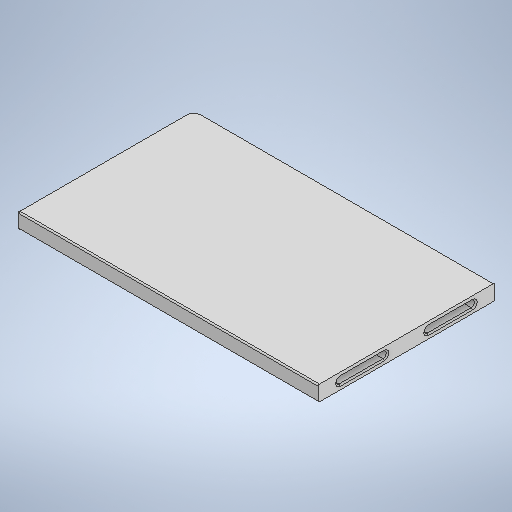
# Autodesk Inventor part: RighClamo3
Saved by Autodesk Inventor 2025.3 (Build 293356000, 356)
## iProperties
Created: 2025-11-20
Part Number: RighClamo3
Material: Generic
Document SubType Name: Modeling
Designer: User
Density: 1 g/cm^3
Appearance: Default
Author: User
Autodesk Inventor part; units mm, degrees
ref_plane "YZ Plane" through (0, 0, 0) normal (1, 0, 0) x (0, 1, 0)
ref_plane "XZ Plane" through (0, 0, 0) normal (0, 1, 0) x (-1, 0, 0)
ref_plane "XY Plane" through (0, 0, 0) normal (0, 0, 1) x (1, 0, 0)
sketch "Sketch1" plane through (0, 0, 0) normal (0, 1, 0) x (-1, 0, 0)
  line L0 (0, 0) -> (420, 0)
  line L1 (420, 0) -> (420, -40)
  line L2 (420, -40) -> (0, -40)
  line L3 (0, -40) -> (0, 0)
  dimension "d0" = 420
  dimension "d1" = 40
  constraints: 8 end point, 2 parallel, 1 horizontal, 1 perpendicular
  measures "d0" distance of L1.end L2.end
  measures "d1" distance of L0.end L1.end
extrude "Extrusion1" add sketch "Sketch1" along normal blind 3.5
fillet "Fillet1" radius 0.3 10 edges at (-210, 3.5, 0) (-210, 0, 0) (0, 0, -20) (0, 3.5, -20) (0, 1.75, -40) (-210, 3.5, -40) (-210, 0, -40) (-420, 0, -20) (-420, 1.75, -40) (-420, 3.5, -20)
sketch "Sketch2" plane through (0, 0, 0) normal (0, -1, 0) x (1, 0, 0)
  line L0 (-419.7, -39.7) -> (-419.7, -0.3) projected
  line L1 (-419.7, -20) -> (0, -20)
  circle A0 centre (-405, -20) radius 5
  circle A1 centre (-375, -20) radius 5
  circle A2 centre (-345, -20) radius 5
  circle A3 centre (-315, -20) radius 5
  line L2 (-420, 0) -> (-420, -39.7) projected
  line L3 (-315, -20) -> (-315, -8.0411)
  line L4 (-210.3, -20) -> (-630, -20)
  circle A4 centre (-225, -20) radius 5
  circle A5 centre (-255, -20) radius 5
  circle A6 centre (-285, -20) radius 5
  point P0 (0, 0)
  point P1 (-420, -0.3)
  dimension "d5" = 10
  dimension "d6" = 10
  dimension "d7" = 10
  dimension "d8" = 10
  dimension "d9" = 15
  dimension "d10" = 30
  dimension "d11" = 30
  dimension "d12" = 30
  constraints: 7 centre point, 7 point on line, 6 end point, 5 symmetric about line, 1 horizontal, 1 midpoint, 1 vertical, 3 other
  measures "d5" diameter of A0
  measures "d6" diameter of A1
  measures "d7" diameter of A2
  measures "d8" diameter of A3
  measures "d9" distance from line of L2 A0.centre
  measures "d10" distance of A1.centre A0.centre
  measures "d11" distance of A2.centre A1.centre
  measures "d12" distance of L3.start A2.centre
ref_plane "Work Plane1" through (-210, 0.3, -39.7) normal (1, 0, 0) x (0, 0, -1)
extrude "Extrusion2" cut sketch "Sketch2" against normal blind 3
mirror "Mirror1" about plane through (-210, 0.3, -39.7) normal (1, 0, 0) of "Extrusion2"
fillet "Fillet2" radius 2 6 edges at (-0.0879, 3.4121, -0.0879) (-0.0879, 0.0879, -0.0879) (0, 1.75, 0) (-419.9121, 3.4121, -0.0879) (-419.9121, 0.0879, -0.0879) (-420, 1.75, 0)
ref_plane "Work Plane2" through (-418, 0.3, -20) normal (0, 0, 1) x (1, 0, 0)
mirror "Mirror2" about plane through (-418, 0.3, -20) normal (0, 0, 1) remove original yes
sketch "Sketch3" plane through (-419.7, 3.5, -0.3) normal (0, 1, 0) x (1, 0, 0)
  line L0 (427.9018, 74.6307) -> (247.9018, 74.6307)
  line L1 (247.9018, 74.6307) -> (247.9018, -47.3259)
  line L2 (247.9018, -47.3259) -> (427.9018, -47.3259)
  line L3 (427.9018, -47.3259) -> (427.9018, 74.6307)
  line L4 (247.9018, 74.6307) -> (67.9018, 74.6307)
  line L5 (67.9018, 74.6307) -> (67.9018, -51.3741)
  line L6 (67.9018, -51.3741) -> (247.9018, -51.3741)
  line L7 (247.9018, -51.3741) -> (247.9018, 74.6307)
  line L8 (67.9018, 74.6307) -> (-27.6852, 74.6307)
  line L9 (-27.6852, 74.6307) -> (-27.6852, -51.3741)
  line L10 (-27.6852, -51.3741) -> (67.9018, -51.3741)
  line L11 (67.9018, -51.3741) -> (67.9018, 74.6307)
  point P0 (419.7, -0.3)
  point P1 (247.9018, -47.3259)
  point P2 (67.9018, -51.3741)
  point P3 (247.9018, -47.3259)
  dimension "d19" = 180
  dimension "d32" = 180
  constraints: 24 end point, 6 parallel, 3 horizontal, 3 perpendicular, 1 vertical
  measures "d19" distance of L0.start L0.end
  measures "d32" distance between parallel lines of L1 L5
extrude "Extrusion8" cut sketch "Sketch3" against normal through all contours L3 L2 L1 L0 | L1 L7 L6 L5 L4
sketch "Sketch7" plane through (-351.7982, 3.5, -0.3) normal (1, 0, 0) x (0, 0, -1)
  line L0 (4.7, -1.75) -> (14.7, -1.75) construction
  line L1 (4.7, -2.5) -> (14.7, -2.5)
  line L2 (14.7, -1) -> (4.7, -1)
  arc A0 (4.7, -1) -> (4.7, -2.5) centre (4.7, -1.75) ccw
  arc A1 (14.7, -2.5) -> (14.7, -1) centre (14.7, -1.75) ccw
  line L3 (24.7, -1.75) -> (34.7, -1.75) construction
  line L4 (24.7, -2.5) -> (34.7, -2.5)
  line L5 (34.7, -1) -> (24.7, -1)
  arc A2 (24.7, -1) -> (24.7, -2.5) centre (24.7, -1.75) ccw
  arc A3 (34.7, -2.5) -> (34.7, -1) centre (34.7, -1.75) ccw
  line L6 (39.7, -0.3) -> (39.7, -3.2) projected
  line L7 (-0.3, -3.2) -> (-0.3, -0.3) projected
  point P0 (-0.3, -3.5)
  point P1 (9.7, -1.75)
  point P2 (29.7, -1.75)
  dimension "d55" = 5
  dimension "d56" = 1.5
  dimension "d57" = 5
  dimension "d58" = 1.5
  dimension "d59" = 10
  dimension "d60" = 10
  constraints: 16 end point, 8 point on circle, 8 tangent, 4 centre point, 2 horizontal, 2 midpoint, 2 parallel
  measures "d55" distance of point (9.7, -1.75) L0.end
  measures "d56" diameter of A1
  measures "d57" distance of point (29.7, -1.75) L3.end
  measures "d58" diameter of A3
  measures "d59" distance from line of L6 point (29.7, -1.75)
  measures "d60" distance from line of L7 point (9.7, -1.75)
extrude "Extrusion9" cut sketch "Sketch7" against normal blind 16
chamfer "Chamfer3" distance 0.3 angle 45 8 edges at (-351.7982, 1.75, -15.75) (-351.7982, 1, -10) (-351.7982, 1.75, -4.25) (-351.7982, 2.5, -10) (-351.7982, 1.75, -24.25) (-351.7982, 2.5, -30) (-351.7982, 1.75, -35.75) (-351.7982, 1, -30)
body "Solid1"
